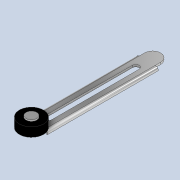
# Autodesk Inventor part: High Voltage Limit Switch Arm
Saved by Autodesk Inventor 2022 (Build 260153000, 153)
## iProperties
Created: 2021-10-24
Part Number: High Voltage Limit Switch Arm
Material: Generic
Document SubType Name: Modeling
Designer: Coy
Density: 1 g/cm^3
Appearance: Chrome - Polished
Author: Coy
Autodesk Inventor part; units mm, degrees
ref_plane "YZ Plane" through (0, 0, 0) normal (1, 0, 0) x (0, 1, 0)
ref_plane "XZ Plane" through (0, 0, 0) normal (0, 1, 0) x (-1, 0, 0)
sketch "Sketch1" plane through (0, 0, 0) normal (0, 1, 0) x (-1, 0, 0)
  circle A0 centre (0, 0) radius 6
  line L0 (0, 0) -> (0, 90) construction
  circle A1 centre (0, 90) radius 6
  line L1 (12.9035, -6) -> (-17.4473, -6) construction
  line L2 (12.9035, 96) -> (-17.4473, 96) construction
  line L3 (6, 90) -> (6, 0)
  line L4 (-6, 90) -> (-6, 0)
  line L5 (12.9035, 10) -> (-17.4473, 10) construction
  line L6 (12.7918, 80) -> (-17.559, 80) construction
  circle A2 centre (0, 77.5) radius 2.5
  circle A3 centre (0, 12.5) radius 2.5
  line L7 (2.5, 77.5) -> (2.5, 12.5)
  line L8 (-2.5, 12.5) -> (-2.5, 77.5)
  dimension "d0" = 12
  dimension "d1" = 12
  dimension "d2" = 102
  dimension "d3" = 70
  dimension "d4" = 16
  dimension "d5" = 5
  dimension "d6" = 5
  constraints: 18 end point, 11 tangent, 8 point on circle, 4 centre point, 4 horizontal, 2 coincident, 2 point on line, 1 vertical
  measures "d0" diameter of A0
  measures "d1" diameter of A1
  measures "d2" distance between parallel lines of L2 L1
  measures "d3" distance between parallel lines of L5 L6
  measures "d4" distance between parallel lines of L1 L5
  measures "d5" diameter of A2
  measures "d6" diameter of A3
extrude "Extrusion1" add sketch "Sketch1" along normal blind 1.5
ref_plane "Work Plane2" through (6, 0, 86) normal (0, 0, 1) x (0, 1, 0)
ref_plane "Work Plane1" through (6, 0, 90) normal (0, 0, 1) x (0, 1, 0)
sketch "Sketch2" plane through (6, 0, 86) normal (0, 0, 1) x (0, 1, 0)
  line L0 (1.5, 0) -> (1.5, 12) projected
  line L1 (-1.5, -2.125) -> (1.5, -2.125) construction
  line L2 (1.5, -2.125) -> (1.5, 14.125) construction
  line L3 (1.5, 14.125) -> (-1.5, 14.125) construction
  line L4 (-1.5, 14.125) -> (-1.5, -2.125) construction
  line L5 (0, 12) -> (1.5, 12) projected
  line L6 (0, 12) -> (0, 0) projected
  line L7 (0, 0) -> (1.5, 0) projected
  line L8 (1.5, 12) -> (1.5, 0) projected
  line L9 (0, 12) -> (1.5, 12) projected
  arc A0 (1.5, 12) -> (-0.9425, 14.125) centre (-0.6456, 12) ccw
  arc A1 (0, 12) -> (-1.5, 13.5675) centre (-1.569, 12) ccw
  line L10 (-1.5, 13.5675) -> (-0.9425, 14.125)
  line L11 (0, 0) -> (0, 12) projected
  line L12 (0, 6) -> (-3.8255, 6) construction
  arc A2 (-0.9425, -2.125) -> (1.5, 0) centre (-0.6456, 0) ccw
  arc A3 (-1.5, -1.5675) -> (0, 0) centre (-1.569, 0) ccw
  line L13 (-1.5, -1.5675) -> (-0.9425, -2.125)
  dimension "d11" = 3
  dimension "d12" = 16.25
  dimension "d13" = 2.125
  dimension "d15" = 1.5
  dimension "d16" = 45
  constraints: 14 end point, 8 point on circle, 6 symmetric about line, 4 centre point, 3 tangent, 2 horizontal, 2 parallel, 2 point on line, 1 perpendicular, 2 other
  measures "d11" distance of L2.end L3.end
  measures "d12" distance of L3.end L1.start
  measures "d13" distance between parallel lines of L5 L3
  measures "d15" distance between parallel lines of L6 L2
  measures "d16" angle of L4 L10
extrude "Extrusion2" add sketch "Sketch2" against normal blind 82 contours A2 L13 A3 L7 | L5 A1 L10 A0
sketch "Sketch3" plane through (0, 1.5, 0) normal (0, 1, 0) x (1, 0, 0)
  arc A0 (-6, -90) -> (6, -90) centre (0, -90) ccw projected
  circle A1 centre (0, -90) radius 9
  point P0 (0, 0)
  dimension "d19" = 18
  constraints: 1 centre point, 1 coincident
  measures "d19" diameter of A1
extrude "Extrusion3" add sketch "Sketch3" along normal blind 6.75
sketch "Sketch4" plane through (0, 8.25, 90) normal (0, 1, 0) x (1, 0, 0)
  circle A0 centre (0, 0) radius 4
  point P0 (0, 90)
  dimension "d22" = 8
  constraints: 1 centre point
  measures "d22" diameter of A0
extrude "Extrusion4" add sketch "Sketch4" along normal blind 1
equation "\"d1\" = d0"
equation "\"d6\" = d5"
body "Solid1"
